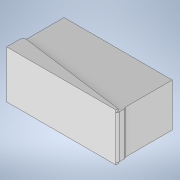
# Autodesk Inventor part: Ammo-Item-Medium
Saved by Autodesk Inventor 2020 (Build 240168000, 168)
## iProperties
Created: 2019-09-20
Part Number: Ammo-Item-Medium
Material: Generic
Document SubType Name: Modeling
Designer: vifly_01
Density: 1 g/cm^3
Appearance: Default
Author: vifly_01
Autodesk Inventor part; units mm, degrees
ref_plane "YZ Plane" through (0, 0, 0) normal (1, 0, 0) x (0, 1, 0)
ref_plane "XZ Plane" through (0, 0, 0) normal (0, 1, 0) x (-1, 0, 0)
ref_plane "XY Plane" through (0, 0, 0) normal (0, 0, 1) x (1, 0, 0)
sketch "Sketch1" plane through (0, 0, 0) normal (0, 0, 1) x (1, 0, 0)
  line L0 (-25, -10) -> (25, -10)
  line L1 (25, -10) -> (25, 10)
  line L2 (25, 10) -> (-25, 10)
  line L3 (-25, 10) -> (-25, -10)
  line L4 (-25, -10) -> (25, 10) construction
  line L5 (25, -10) -> (-25, 10) construction
  point P0 (0, 0)
  dimension "d0" = 50
  dimension "d1" = 20
  constraints: 12 end point, 2 midpoint, 2 parallel, 1 horizontal, 1 perpendicular
  measures "d0" distance of L2.end L1.end
  measures "d1" distance of L1.end L0.end
extrude "Extrusion1" add sketch "Sketch1" along normal blind 25
sketch "Sketch3" plane through (-25, -10, 0) normal (0, -1, 0) x (1, 0, 0)
  line L0 (0, 26) -> (50, 26)
  line L1 (50, 26) -> (50, 25)
  line L2 (50, 0) -> (50, 25) projected
  line L3 (50, 25) -> (1.2607, 18.4598)
  line L4 (0, 25) -> (50, 25) projected
  line L5 (0, 25) -> (50, 25)
  line L6 (0, 25) -> (-0.5, 25)
  line L7 (0, 26) -> (-0.5, 26)
  line L8 (-0.5, 26) -> (-0.5, 25)
  line L9 (-0.5, 25) -> (-0.5, 20)
  arc A0 (-0.5, 20) -> (1.2607, 18.4598) centre (1.054, 20) ccw
  point P0 (25, 0)
  dimension "d4" = 1
  dimension "d6" = 48.7393
  dimension "d12" = 0.5
  dimension "d13" = 5
  constraints: 16 end point, 2 horizontal, 2 perpendicular, 2 point on circle, 2 tangent, 1 centre point, 1 point on line, 1 vertical
  measures "d4" distance of L4.start L0.start
  measures "d6" horizontal distance of L1.end L3.end
  measures "d12" distance of L4.start L6.end
  measures "d13" distance of L6.end L9.end
extrude "Extrusion2" add sketch "Sketch3" along normal blind 1
extrude "Extrusion3" add sketch "Sketch3" against normal blind 21
sketch "Sketch4" plane through (-25.5, -11, 20) normal (-1, 0, 0) x (0, 0, 1)
  line L0 (-1.5402, 21) -> (5, 21) projected
  line L1 (5, 21) -> (-1.5402, 21)
  line L2 (-1.5402, 1) -> (-1.5402, 0) projected
  line L3 (-1.5402, 21) -> (-1.5402, 1)
  line L4 (-20, 1) -> (5, 1) projected
  line L5 (-1.5402, 1) -> (5, 1)
  line L6 (5, 1) -> (5, 21)
  point P0 (-20, 11)
  constraints: 8 end point, 2 collinear, 2 perpendicular
extrude "Extrusion4" cut sketch "Sketch4" against normal blind 0.5
sketch "Sketch5" plane through (25, -10, 0) normal (1, 0, 0) x (0, 0, -1)
  line L0 (-25, 0) -> (-18.4598, 0) projected
  line L1 (-18.4598, 20) -> (-25, 20) projected
  line L2 (-21.7299, 0) -> (-21.7299, 20)
  line L3 (-21.7299, 20) -> (-25, 20)
  line L4 (-25, 20) -> (-25, 0)
  line L5 (-25, 0) -> (-21.7299, 0)
  point P0 (0, 10)
  constraints: 8 end point, 2 midpoint, 2 parallel, 1 perpendicular
extrude "Extrusion5" add sketch "Sketch5" along normal blind 0.5
sketch "Sketch6" plane through (-25, -10, 0) normal (0, -1, 0) x (1, 0, 0)
  line L0 (50, 25) -> (50.5, 25) projected
  line L1 (50, 25) -> (50, 26) projected
  arc A0 (50.5, 25) -> (50, 26) centre (49.3829, 25.0664) ccw
  point P0 (25, 0)
  constraints: 2 point on circle, 1 centre point
extrude "Extrusion6" add sketch "Sketch6" against normal blind 20
sketch "Sketch7" plane through (-25, -10, 0) normal (0, -1, 0) x (1, 0, 0)
  line L0 (50, 21.7299) -> (50.5, 21.7299) projected
  line L1 (50, 21.7299) -> (50.5, 22.5959)
  line L2 (50.5, 21.7299) -> (50.5, 25) projected
  line L3 (50, 0) -> (50, 21.7299) projected
  line L4 (50, 21.7299) -> (50.5, 21.7299)
  line L5 (50.5, 21.7299) -> (50.5, 22.5959)
  point P0 (25, 0)
  dimension "d20" = 1
  constraints: 6 end point, 2 collinear, 1 point on line
  measures "d20" distance of L0.start L1.end
extrude "Extrusion7" cut sketch "Sketch7" against normal blind 20
body "Solid1"
